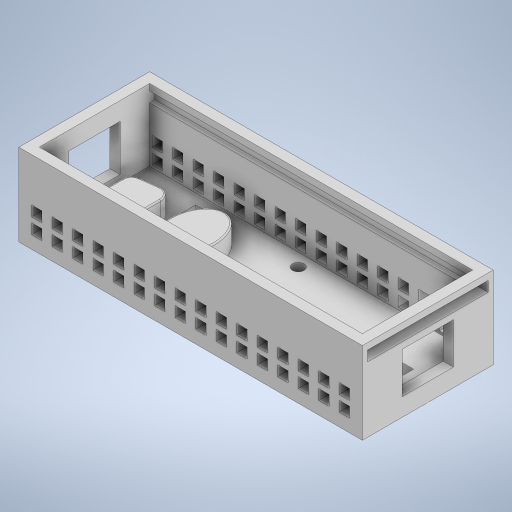
# Autodesk Inventor part: Milestone3
Saved by Autodesk Inventor 2024 (Build 280153000, 153)
## iProperties
Created: 2023-11-12
Part Number: Milestone3
Material: Generic
Document SubType Name: Modeling
Designer: Yuvraj
Density: 1 g/cm^3
Appearance: Default
Author: Yuvraj
Autodesk Inventor part; units mm, degrees
ref_plane "YZ Plane" through (0, 0, 0) normal (1, 0, 0) x (0, 1, 0)
ref_plane "XZ Plane" through (0, 0, 0) normal (0, 1, 0) x (-1, 0, 0)
ref_plane "XY Plane" through (0, 0, 0) normal (0, 0, 1) x (1, 0, 0)
sketch "Sketch1" plane through (0, 0, 0) normal (0, 1, 0) x (-1, 0, 0)
  line L0 (67, 25.5) -> (-67, 25.5)
  line L1 (-67, 25.5) -> (-67, -25.5)
  line L2 (-67, -25.5) -> (67, -25.5)
  line L3 (67, -25.5) -> (67, 25.5)
  point P0 (0, 0)
  dimension "d0" = 25.5
  dimension "d1" = 67
  dimension "d2" = 67
  dimension "d3" = 25.5
  constraints: 8 end point, 2 parallel, 1 horizontal, 1 perpendicular
  measures "d0" distance from line of point (0, 0) L0
  measures "d1" distance from line of point (0, 0) L3
  measures "d2" distance from line of L1 point (0, 0)
  measures "d3" distance from line of L2 point (0, 0)
extrude "Extrusion1" add sketch "Sketch1" along normal blind 32
shell "Shell1" thickness 4 removed faces 1 at (22.3333, 32, -8.5)
sketch "Sketch2" plane through (-63, 4, -21.5) normal (0, 1, 0) x (1, 0, 0)
  line L0 (6.8, -23.6242) -> (6.8, -17.3758)
  line L1 (0, -43) -> (0, 0) projected
  line L2 (21.5, -23.763) -> (21.5, -17.237)
  line L3 (126, -43) -> (0, -43) projected
  line L4 (16.6158, -28.0231) -> (9.8245, -27.0918)
  line L5 (9.8245, -13.9082) -> (16.6158, -12.9769)
  arc A0 (6.8, -23.6242) -> (9.8245, -27.0918) centre (10.3, -23.6242) ccw
  arc A1 (9.8245, -13.9082) -> (6.8, -17.3758) centre (10.3, -17.3758) ccw
  arc A2 (16.6158, -28.0231) -> (21.5, -23.763) centre (17.2, -23.763) ccw
  arc A3 (21.5, -17.237) -> (16.6158, -12.9769) centre (17.2, -17.237) ccw
  point P0 (63, -21.5)
  point P1 (6.8, -26.677)
  point P2 (6.8, -14.323)
  point P3 (6.8, -20.5)
  point P4 (21.5, -20.5)
  dimension "d7" = 6.8
  dimension "d8" = 21.5
  dimension "d9" = 12.354
  dimension "d30" = 22.5
  dimension "d31" = 22.5
  dimension "d34" = 3.5
  dimension "d35" = 4.3
  dimension "d36" = 6.5259
  constraints: 8 end point, 8 point on circle, 8 tangent, 4 centre point, 4 point on line, 2 equal radius, 2 midpoint, 2 vertical
  measures "d7" distance between parallel lines of L0 L1
  measures "d8" distance between parallel lines of L2 L1
  measures "d9" distance of point (6.8, -26.677) point (6.8, -14.323)
  measures "d30" distance from line of L3 point (6.8, -20.5)
  measures "d31" distance from line of L3 point (21.5, -20.5)
  measures "d34" radius of A0
  measures "d35" radius of A2
  measures "d36" distance of L2.start L2.end
sketch "Sketch3" plane through (-63, 4, -21.5) normal (0, 1, 0) x (1, 0, 0)
  line L0 (-8.0993, -247.9931) -> (-17.4532, -247.9931)
  line L1 (-2.142, -242.708) -> (0.2238, -222.9931)
  line L2 (-23.4105, -242.708) -> (-25.7762, -222.9931)
  line L3 (-18.7762, -200.9931) -> (-18.7762, -154.9931)
  line L4 (-18.7762, -154.9931) -> (-22.7762, -152.9931)
  line L5 (-22.7762, -152.9931) -> (-22.7762, -144.9931)
  line L6 (-22.7762, -144.9931) -> (-2.7762, -144.9931)
  line L7 (-2.7762, -144.9931) -> (-2.7762, -152.9931)
  line L8 (-2.7762, -152.9931) -> (-6.7762, -154.9931)
  ellipse E0 centre (-12.7762, -213.6834) end of major axis (-12.7762, -227.1434) minor radius 18
  ellipse E1 centre (-12.7762, -213.6834) end of major axis (-12.7762, -222.6834) minor radius 14
  arc A0 (-8.0993, -247.9931) -> (-2.142, -242.708) centre (-8.0993, -241.9931) ccw
  arc A1 (-23.4105, -242.708) -> (-17.4532, -247.9931) centre (-17.4532, -241.9931) ccw
  arc A2 (-20.0324, -243.5254) -> (-17.4532, -244.9931) centre (-17.4532, -241.9931) ccw
  line L9 (-17.4532, -244.9931) -> (-8.0993, -244.9931)
  arc A3 (-8.0993, -244.9931) -> (-5.5201, -243.5254) centre (-8.0993, -241.9931) ccw
  line L10 (-5.5201, -243.5254) -> (-3.7762, -228.9931)
  line L11 (-3.7762, -228.9931) -> (-21.7762, -228.9931)
  line L12 (-21.7762, -228.9931) -> (-20.0324, -243.5254)
  line L13 (-6.7762, -154.9931) -> (-6.7762, -200.9931)
  line L14 (-21.2493, -249.0332) -> (24.8211, -119.6553)
  point P0 (63, -21.5)
  point P1 (-2.7762, -247.9931)
  point P2 (-22.7762, -247.9931)
  point P3 (-21.2493, -249.0332)
  point P4 (24.8211, -119.6553)
  dimension "d18" = 14
  dimension "d19" = 9
  dimension "d20" = 18
  dimension "d10" = 20
  dimension "d11" = 103
  dimension "d12" = 8
  dimension "d13" = 20
  dimension "d14" = 2
  dimension "d15" = 4
  dimension "d16" = 4
  dimension "d17" = 25
  dimension "d21" = 6
  dimension "d22" = 3
  dimension "d23" = 18
  dimension "d24" = 9
  dimension "d25" = 16
  dimension "d26" = 46
  dimension "d27" = 6
  dimension "d28" = 13
  dimension "d29" = 13
  constraints: 28 end point, 8 point on circle, 4 centre point, 4 equal length, 4 point on line, 4 tangent, 2 coincident, 2 horizontal, 2 parallel, 2 perpendicular, 2 vertical, 1 equal radius, 13 other
  measures "d10" distance of point (-2.776, -247.993) point (-22.776, -247.993)
  measures "d11" distance between parallel lines of L6 L0
  measures "d12" distance of L6.end L7.end
  measures "d13" distance of L5.end L6.end
  measures "d14" vertical distance of L3.end L4.end
  measures "d15" horizontal distance of L3.end L4.end
  measures "d16" horizontal distance of L7.end L8.end
  measures "d17" distance from line of L1.end L0
  measures "d21" radius of A0
  measures "d22" distance between parallel lines of L0 L9
  measures "d23" distance of L10.end L11.end
  measures "d24" horizontal distance of point (-12.776, -213.683) L10.end
  measures "d25" distance between parallel lines of L11 L9
  measures "d26" distance of L8.end L13.end
  measures "d27" distance from line of point (-12.776, -213.683) L13
  measures "d28" horizontal distance of point (-12.776, -213.683) L1.end
extrude "Extrusion2" add sketch "Sketch2" along normal blind 8
fillet "Fillet1" radius 0.5 8 edges at (-49.7799, 12, -8.0574) (-55.3376, 12, -6.4248) (-56.2, 12, -1) (-55.3376, 12, 4.4248) (-49.7799, 12, 6.0574) (-42.9735, 12, 5.5035) (-41.5, 12, -1) (-42.9735, 12, -7.5035)
sketch "Sketch4" plane through (-63, 4, -21.5) normal (0, 1, 0) x (1, 0, 0)
  ellipse E0 centre (38, -21.5) end of major axis (38, -34.2) minor radius 8.7
  line L0 (126, -43) -> (0, -43) projected
  line L1 (21.5, -17.237) -> (21.5, -23.763) projected
  point P0 (63, -21.5)
  dimension "d41" = 21.5
  dimension "d42" = 12.7
  dimension "d43" = 8.7
  dimension "d44" = 16.5
  constraints: 1 centre point, 1 other
  measures "d41" distance from line of L0 E0.centre
  measures "d44" distance from line of L1 E0.centre
extrude "Extrusion3" add sketch "Sketch4" along normal blind 8
fillet "Fillet2" radius 0.5 1 edges at (-25, 12, -12.7)
sketch "Sketch6" plane through (-67, 0, 25.5) normal (0, 0, 1) x (1, 0, 0)
  line L0 (5, 5) -> (9, 5)
  line L1 (9, 5) -> (9, 9)
  line L2 (9, 9) -> (5, 9)
  line L3 (5, 9) -> (5, 5)
  line L4 (0, 0) -> (0, 32) projected
  line L5 (0, 0) -> (134, 0) projected
  line L6 (17, 5) -> (17, 9)
  line L7 (13, 5) -> (17, 5)
  line L8 (13, 9) -> (13, 5)
  line L9 (17, 9) -> (13, 9)
  line L10 (25, 5) -> (25, 9)
  line L11 (21, 5) -> (25, 5)
  line L12 (21, 9) -> (21, 5)
  line L13 (25, 9) -> (21, 9)
  line L14 (33, 5) -> (33, 9)
  line L15 (29, 5) -> (33, 5)
  line L16 (29, 9) -> (29, 5)
  line L17 (33, 9) -> (29, 9)
  line L18 (41, 5) -> (41, 9)
  line L19 (37, 5) -> (41, 5)
  line L20 (37, 9) -> (37, 5)
  line L21 (41, 9) -> (37, 9)
  line L22 (49, 5) -> (49, 9)
  line L23 (45, 5) -> (49, 5)
  line L24 (45, 9) -> (45, 5)
  line L25 (49, 9) -> (45, 9)
  line L26 (57, 5) -> (57, 9)
  line L27 (53, 5) -> (57, 5)
  line L28 (53, 9) -> (53, 5)
  line L29 (57, 9) -> (53, 9)
  line L30 (65, 5) -> (65, 9)
  line L31 (61, 5) -> (65, 5)
  line L32 (61, 9) -> (61, 5)
  line L33 (65, 9) -> (61, 9)
  line L34 (73, 5) -> (73, 9)
  line L35 (69, 5) -> (73, 5)
  line L36 (69, 9) -> (69, 5)
  line L37 (73, 9) -> (69, 9)
  line L38 (81, 5) -> (81, 9)
  line L39 (77, 5) -> (81, 5)
  line L40 (77, 9) -> (77, 5)
  line L41 (81, 9) -> (77, 9)
  line L42 (89, 5) -> (89, 9)
  line L43 (85, 5) -> (89, 5)
  line L44 (85, 9) -> (85, 5)
  line L45 (89, 9) -> (85, 9)
  line L46 (97, 5) -> (97, 9)
  line L47 (93, 5) -> (97, 5)
  line L48 (93, 9) -> (93, 5)
  line L49 (97, 9) -> (93, 9)
  line L50 (105, 5) -> (105, 9)
  line L51 (101, 5) -> (105, 5)
  line L52 (101, 9) -> (101, 5)
  line L53 (105, 9) -> (101, 9)
  line L54 (113, 5) -> (113, 9)
  line L55 (109, 5) -> (113, 5)
  line L56 (109, 9) -> (109, 5)
  line L57 (113, 9) -> (109, 9)
  line L58 (121, 5) -> (121, 9)
  line L59 (117, 5) -> (121, 5)
  line L60 (117, 9) -> (117, 5)
  line L61 (121, 9) -> (117, 9)
  line L62 (129, 5) -> (129, 9)
  line L63 (125, 5) -> (129, 5)
  line L64 (125, 9) -> (125, 5)
  line L65 (129, 9) -> (125, 9)
  line L66 (9, 11) -> (9, 15)
  line L67 (5, 11) -> (9, 11)
  line L68 (5, 15) -> (5, 11)
  line L69 (9, 15) -> (5, 15)
  line L70 (17, 11) -> (17, 15)
  line L71 (13, 11) -> (17, 11)
  line L72 (13, 15) -> (13, 11)
  line L73 (17, 15) -> (13, 15)
  line L74 (25, 11) -> (25, 15)
  line L75 (21, 11) -> (25, 11)
  line L76 (21, 15) -> (21, 11)
  line L77 (25, 15) -> (21, 15)
  line L78 (33, 11) -> (33, 15)
  line L79 (29, 11) -> (33, 11)
  line L80 (29, 15) -> (29, 11)
  line L81 (33, 15) -> (29, 15)
  line L82 (41, 11) -> (41, 15)
  line L83 (37, 11) -> (41, 11)
  line L84 (37, 15) -> (37, 11)
  line L85 (41, 15) -> (37, 15)
  line L86 (49, 11) -> (49, 15)
  line L87 (45, 11) -> (49, 11)
  line L88 (45, 15) -> (45, 11)
  line L89 (49, 15) -> (45, 15)
  line L90 (57, 11) -> (57, 15)
  line L91 (53, 11) -> (57, 11)
  line L92 (53, 15) -> (53, 11)
  line L93 (57, 15) -> (53, 15)
  line L94 (65, 11) -> (65, 15)
  line L95 (61, 11) -> (65, 11)
  line L96 (61, 15) -> (61, 11)
  line L97 (65, 15) -> (61, 15)
  line L98 (73, 11) -> (73, 15)
  line L99 (69, 11) -> (73, 11)
  line L100 (69, 15) -> (69, 11)
  line L101 (73, 15) -> (69, 15)
  line L102 (81, 11) -> (81, 15)
  line L103 (77, 11) -> (81, 11)
  line L104 (77, 15) -> (77, 11)
  line L105 (81, 15) -> (77, 15)
  line L106 (89, 11) -> (89, 15)
  line L107 (85, 11) -> (89, 11)
  line L108 (85, 15) -> (85, 11)
  line L109 (89, 15) -> (85, 15)
  line L110 (97, 11) -> (97, 15)
  line L111 (93, 11) -> (97, 11)
  line L112 (93, 15) -> (93, 11)
  line L113 (97, 15) -> (93, 15)
  line L114 (105, 11) -> (105, 15)
  line L115 (101, 11) -> (105, 11)
  line L116 (101, 15) -> (101, 11)
  line L117 (105, 15) -> (101, 15)
  line L118 (113, 11) -> (113, 15)
  line L119 (109, 11) -> (113, 11)
  line L120 (109, 15) -> (109, 11)
  line L121 (113, 15) -> (109, 15)
  line L122 (121, 11) -> (121, 15)
  line L123 (117, 11) -> (121, 11)
  line L124 (117, 15) -> (117, 11)
  line L125 (121, 15) -> (117, 15)
  line L126 (129, 11) -> (129, 15)
  line L127 (125, 11) -> (129, 11)
  line L128 (125, 15) -> (125, 11)
  line L129 (129, 15) -> (125, 15)
  point P0 (67, 0)
  point P1 (5, 7)
  point P2 (9, 7)
  point P3 (7, 5)
  point P4 (7, 9)
  point P5 (17, 7)
  point P6 (15, 5)
  point P7 (13, 7)
  point P8 (15, 9)
  point P9 (25, 7)
  point P10 (23, 5)
  point P11 (21, 7)
  point P12 (23, 9)
  point P13 (33, 7)
  point P14 (31, 5)
  point P15 (29, 7)
  point P16 (31, 9)
  point P17 (41, 7)
  point P18 (39, 5)
  point P19 (37, 7)
  point P20 (39, 9)
  point P21 (49, 7)
  point P22 (47, 5)
  point P23 (45, 7)
  point P24 (47, 9)
  point P25 (57, 7)
  point P26 (55, 5)
  point P27 (53, 7)
  point P28 (55, 9)
  point P29 (65, 7)
  point P30 (63, 5)
  point P31 (61, 7)
  point P32 (63, 9)
  point P33 (73, 7)
  point P34 (71, 5)
  point P35 (69, 7)
  point P36 (71, 9)
  point P37 (81, 7)
  point P38 (79, 5)
  point P39 (77, 7)
  point P40 (79, 9)
  point P41 (89, 7)
  point P42 (87, 5)
  point P43 (85, 7)
  point P44 (87, 9)
  point P45 (97, 7)
  point P46 (95, 5)
  point P47 (93, 7)
  point P48 (95, 9)
  point P49 (105, 7)
  point P50 (103, 5)
  point P51 (101, 7)
  point P52 (103, 9)
  point P53 (113, 7)
  point P54 (111, 5)
  point P55 (109, 7)
  point P56 (111, 9)
  point P57 (121, 7)
  point P58 (119, 5)
  point P59 (117, 7)
  point P60 (119, 9)
  point P61 (129, 7)
  point P62 (127, 5)
  point P63 (125, 7)
  point P64 (127, 9)
  point P65 (9, 13)
  point P66 (7, 11)
  point P67 (5, 13)
  point P68 (7, 15)
  point P69 (17, 13)
  point P70 (15, 11)
  point P71 (13, 13)
  point P72 (15, 15)
  point P73 (25, 13)
  point P74 (23, 11)
  point P75 (21, 13)
  point P76 (23, 15)
  point P77 (33, 13)
  point P78 (31, 11)
  point P79 (29, 13)
  point P80 (31, 15)
  point P81 (41, 13)
  point P82 (39, 11)
  point P83 (37, 13)
  point P84 (39, 15)
  point P85 (49, 13)
  point P86 (47, 11)
  point P87 (45, 13)
  point P88 (47, 15)
  point P89 (57, 13)
  point P90 (55, 11)
  point P91 (53, 13)
  point P92 (55, 15)
  point P93 (65, 13)
  point P94 (63, 11)
  point P95 (61, 13)
  point P96 (63, 15)
  point P97 (73, 13)
  point P98 (71, 11)
  point P99 (69, 13)
  point P100 (71, 15)
  point P101 (81, 13)
  point P102 (79, 11)
  point P103 (77, 13)
  point P104 (79, 15)
  point P105 (89, 13)
  point P106 (87, 11)
  point P107 (85, 13)
  point P108 (87, 15)
  point P109 (97, 13)
  point P110 (95, 11)
  point P111 (93, 13)
  point P112 (95, 15)
  point P113 (105, 13)
  point P114 (103, 11)
  point P115 (101, 13)
  point P116 (103, 15)
  point P117 (113, 13)
  point P118 (111, 11)
  point P119 (109, 13)
  point P120 (111, 15)
  point P121 (121, 13)
  point P122 (119, 11)
  point P123 (117, 13)
  point P124 (119, 15)
  point P125 (129, 13)
  point P126 (127, 11)
  point P127 (125, 13)
  point P128 (127, 15)
  dimension "d59" = 4
  dimension "d60" = 4
  dimension "d61" = 5
  dimension "d62" = 9
  dimension "d65" = 8
  dimension "d68" = 6
  constraints: 256 end point, 4 midpoint, 2 collinear, 2 horizontal, 2 parallel, 1 perpendicular, 1 vertical, 370 other
  measures "d59" distance of point (5, 7) point (9, 7)
  measures "d60" distance of point (7, 5) point (7, 9)
  measures "d61" distance between parallel lines of L4 L3
  measures "d62" distance between parallel lines of L5 L2
  measures "d65" distance of L0.end L6.start
  measures "d68" distance of L0.end L66.start
extrude "Extrusion4" cut sketch "Sketch6" against normal blind 4
sketch "Sketch7" plane through (67, 0, 25.5) normal (1, 0, 0) x (0, 0, -1)
  line L0 (15.5, 7) -> (29.5, 7)
  line L1 (29.5, 7) -> (29.5, 23)
  line L2 (29.5, 23) -> (15.5, 23)
  line L3 (15.5, 23) -> (15.5, 7)
  line L4 (0, 32) -> (51, 32) projected
  line L5 (0, 0) -> (51, 0) projected
  line L6 (0, 0) -> (0, 32) projected
  point P0 (25.5, 0)
  point P1 (22.5, 23)
  dimension "d73" = 9
  dimension "d74" = 7
  dimension "d75" = 15.5
  dimension "d76" = 7
  constraints: 8 end point, 2 parallel, 1 horizontal, 1 midpoint, 1 perpendicular
  measures "d73" distance between parallel lines of L4 L2
  measures "d74" distance between parallel lines of L5 L0
  measures "d75" distance between parallel lines of L6 L3
  measures "d76" distance from line of point (22.5, 23) L1
extrude "Extrusion5" cut sketch "Sketch7" against normal blind 4
sketch "Sketch8" plane through (-67, 0, -25.5) normal (-1, 0, 0) x (0, 0, 1)
  line L0 (21.5, 25) -> (35.5, 25)
  line L1 (35.5, 25) -> (35.5, 7)
  line L2 (35.5, 7) -> (21.5, 7)
  line L3 (21.5, 7) -> (21.5, 25)
  line L4 (51, 0) -> (51, 32) projected
  line L5 (0, 32) -> (51, 32) projected
  line L6 (0, 0) -> (51, 0) projected
  point P0 (25.5, 0)
  point P1 (28.5, 25)
  point P2 (-152.1555, -14.1237)
  dimension "d79" = 15.5
  dimension "d80" = 7
  dimension "d81" = 7
  dimension "d82" = 7
  constraints: 8 end point, 2 parallel, 1 horizontal, 1 midpoint, 1 perpendicular
  measures "d79" distance between parallel lines of L4 L1
  measures "d80" distance between parallel lines of L5 L0
  measures "d81" distance between parallel lines of L6 L2
  measures "d82" distance from line of point (28.5, 25) L3
extrude "Extrusion6" cut sketch "Sketch8" against normal blind 4
mirror "Mirror1" about plane through (0, 0, 0) normal (0, 0, 1) of "Extrusion4", "Extrusion6", "Extrusion5"
sketch "Sketch10" plane through (-63, 4, -21.5) normal (0, 1, 0) x (1, 0, 0)
  line L0 (51, -17) -> (60, -17)
  line L1 (60, -17) -> (60, -26)
  line L2 (60, -26) -> (51, -26)
  line L3 (51, -26) -> (51, -17)
  line L4 (0, 0) -> (126, 0) projected
  line L5 (126, -43) -> (0, -43) projected
  line L6 (0, -43) -> (0, 0) projected
  line L7 (126, 0) -> (126, -43) projected
  line L8 (66, -17) -> (75, -17)
  line L9 (75, -17) -> (75, -26)
  line L10 (75, -26) -> (66, -26)
  line L11 (66, -26) -> (66, -17)
  line L12 (66, -17) -> (75, -17)
  line L13 (75, -17) -> (75, -26)
  line L14 (75, -26) -> (66, -26)
  line L15 (66, -26) -> (66, -17)
  line L16 (81, -17) -> (90, -17)
  line L17 (90, -17) -> (90, -26)
  line L18 (90, -26) -> (81, -26)
  line L19 (81, -26) -> (81, -17)
  line L20 (81, -17) -> (90, -17)
  line L21 (90, -17) -> (90, -26)
  line L22 (90, -26) -> (81, -26)
  line L23 (81, -26) -> (81, -17)
  line L24 (96, -17) -> (105, -17)
  line L25 (105, -17) -> (105, -26)
  line L26 (105, -26) -> (96, -26)
  line L27 (96, -26) -> (96, -17)
  line L28 (96, -17) -> (105, -17)
  line L29 (105, -17) -> (105, -26)
  line L30 (105, -26) -> (96, -26)
  line L31 (96, -26) -> (96, -17)
  line L32 (111, -17) -> (120, -17)
  line L33 (120, -17) -> (120, -26)
  line L34 (120, -26) -> (111, -26)
  line L35 (111, -26) -> (111, -17)
  ellipse E0 centre (38, -21.5) end of major axis (38, -34.2) minor radius 8.7 projected
  line L36 (22, -39) -> (29, -39)
  line L37 (29, -39) -> (29, -30)
  line L38 (29, -30) -> (22, -30)
  line L39 (22, -30) -> (22, -39)
  line L40 (24, -27) -> (28, -27)
  line L41 (28, -27) -> (28, -16)
  line L42 (28, -16) -> (24, -16)
  line L43 (24, -16) -> (24, -27)
  line L44 (22, -13) -> (29, -13)
  line L45 (29, -13) -> (29, -4)
  line L46 (29, -4) -> (22, -4)
  line L47 (22, -4) -> (22, -13)
  point P0 (63, -21.5)
  point P1 (0, -21.5)
  dimension "d99" = 17
  dimension "d100" = 66
  dimension "d101" = 17
  dimension "d102" = 75
  dimension "d105" = 15
  dimension "d108" = 15
  dimension "d134" = 22
  dimension "d135" = 22
  dimension "d136" = 4
  dimension "d137" = 4
  dimension "d138" = 30
  dimension "d139" = 30
  dimension "d140" = 97
  dimension "d141" = 97
  dimension "d142" = 24
  dimension "d143" = 98
  dimension "d144" = 16
  dimension "d145" = 16
  constraints: 88 end point, 8 parallel, 6 horizontal, 4 perpendicular, 2 collinear, 1 midpoint, 54 other
  measures "d99" distance between parallel lines of L4 L0
  measures "d100" distance between parallel lines of L7 L1
  measures "d101" distance between parallel lines of L5 L2
  measures "d102" distance between parallel lines of L7 L3
  measures "d105" distance of L0.start L8.start
  measures "d108" distance of L0.start L12.start
  measures "d134" distance between parallel lines of L6 L39
  measures "d135" distance between parallel lines of L6 L47
  measures "d136" distance between parallel lines of L5 L36
  measures "d137" distance between parallel lines of L4 L46
  measures "d138" distance between parallel lines of L5 L44
  measures "d139" distance between parallel lines of L4 L38
  measures "d140" distance between parallel lines of L7 L37
  measures "d141" distance between parallel lines of L7 L45
  measures "d142" distance between parallel lines of L6 L43
  measures "d143" distance between parallel lines of L7 L41
  measures "d144" distance between parallel lines of L5 L40
  measures "d145" distance between parallel lines of L4 L42
extrude "Extrusion7" cut sketch "Sketch10" against normal blind 4 contours L0 L1 L2 L3 | L8 L9 L10 L11 | L16 L17 L18 L19 | L24 L25 L26 L27 | L32 L33 L34 L35
extrude "Extrusion10" cut sketch "Sketch10" against normal blind 10 contours L39 L38 L37 L36 | L43 L42 L41 L40 | L47 L46 L45 L44
sketch "Sketch15" plane through (67, 0, 25.5) normal (1, 0, 0) x (0, 0, -1)
  point P0 (25.5, 0)
sketch "Sketch16" plane through (67, 0, 25.5) normal (1, 0, 0) x (0, 0, -1)
  line L0 (2, 29.5) -> (49, 29.5)
  line L1 (49, 29.5) -> (49, 25.5)
  line L2 (49, 25.5) -> (2, 25.5)
  line L3 (2, 25.5) -> (2, 29.5)
  line L4 (51, 0) -> (51, 32) projected
  line L5 (0, 0) -> (0, 32) projected
  line L6 (15.5, 23) -> (35.5, 23) projected
  line L7 (0, 32) -> (51, 32) projected
  point P0 (25.5, 0)
  dimension "d166" = 2
  dimension "d167" = 2
  dimension "d168" = 2.5
  dimension "d169" = 2.5
  constraints: 8 end point, 2 parallel, 1 horizontal, 1 perpendicular
  measures "d166" distance between parallel lines of L4 L1
  measures "d167" distance between parallel lines of L5 L3
  measures "d168" distance between parallel lines of L6 L2
  measures "d169" distance between parallel lines of L7 L0
extrude "Extrusion13" cut sketch "Sketch16" against normal blind 130
sketch "Sketch17" plane through (-63, 4, -21.5) normal (0, 1, 0) x (1, 0, 0)
  circle A0 centre (63, -5) radius 2.25
  circle A1 centre (63, -37.512) radius 2.25
  line L0 (130, 4) -> (-4, 4) projected
  line L1 (130, 2) -> (0, 2) projected
  line L2 (130, -45) -> (0, -45) projected
  point P0 (63, -21.5)
  dimension "d172" = 4.5
  dimension "d173" = 4.5
  dimension "d179" = 32.512
  constraints: 2 centre point
  measures "d172" diameter of A1
  measures "d173" diameter of A0
  measures "d179" distance of A1.centre A0.centre
extrude "Extrusion14" cut sketch "Sketch17" against normal blind 10
equation "\"d16\" = d15"
body "Solid1"
